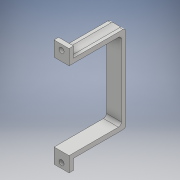
# Autodesk Inventor part: battery-bracket
Saved by Autodesk Inventor 2018 (Build 220112000, 112)
## iProperties
Created: 2017-10-22
Part Number: battery-bracket
Material: Generic
Document SubType Name: Modeling
Designer: leo2a
Density: 1 g/cm^3
Appearance: Default
Author: leo2a
Autodesk Inventor part; units mm, degrees
ref_plane "YZ Plane" through (0, 0, 0) normal (1, 0, 0) x (0, 1, 0)
ref_plane "XZ Plane" through (0, 0, 0) normal (0, 1, 0) x (-1, 0, 0)
ref_plane "XY Plane" through (0, 0, 0) normal (0, 0, 1) x (1, 0, 0)
sketch "Sketch1" plane through (0, 0, 0) normal (1, 0, 0) x (0, 1, 0)
  line L0 (0, 0) -> (0, 26)
  line L1 (0, 26) -> (-35, 26)
  line L2 (0, 0) -> (3, 0)
  line L3 (3, 0) -> (3, 29)
  line L4 (3, 29) -> (-32, 29)
  line L5 (-32, 29) -> (-32, 36)
  line L6 (-32, 36) -> (-35, 36)
  line L7 (-35, 36) -> (-35, 26)
  line L8 (0, 0) -> (0, -26)
  line L9 (0, -26) -> (-35, -26)
  line L10 (3, 0) -> (3, -29)
  line L11 (3, -29) -> (-32, -29)
  line L12 (-32, -29) -> (-32, -36)
  line L13 (-32, -36) -> (-35, -36)
  line L14 (-35, -36) -> (-35, -26)
  dimension "d0" = 26
  dimension "d1" = 35
  dimension "d2" = 3
  dimension "d3" = 29
  dimension "d4" = 35
  dimension "d5" = 7
  constraints: 30 end point, 6 perpendicular, 6 symmetric about line, 1 horizontal, 1 vertical
  measures "d0" distance of L0.start L0.end
  measures "d1" distance of L0.end L1.end
  measures "d2" distance of L0.start L2.end
  measures "d3" distance of L2.end L3.end
  measures "d4" distance of L3.end L4.end
  measures "d5" distance of L4.end L5.end
extrude "Extrusion1" add sketch "Sketch1" along normal blind 10
fillet "Fillet1" radius 2 4 edges at (5, 3, 29) (5, 0, 26) (5, 0, -26) (5, 3, -29)
sketch "Sketch2" plane through (0, -32, 36) normal (0, 1, 0) x (1, 0, 0)
  line L0 (0, 7) -> (0, 0) projected
  line L1 (0, 3.5) -> (5, 3.5)
  line L2 (0, 62) -> (0, 72) projected
  line L3 (0, 72) -> (0, 68.5)
  line L4 (0, 68.5) -> (5, 68.5)
  point P0 (0, 36)
  dimension "d9" = 3.5
  constraints: 6 end point, 2 coincident, 1 horizontal, 1 midpoint, 1 perpendicular, 1 point on line
  measures "d9" distance of L2.end L3.end
hole "Hole1" at (5, -32, 32.5) at (5, -32, -32.5) direction (0, -1, 0) diameter 3.4 end through all clearance for "Socket Head Cap Screw ISO 4762" size "M3" standard "ISO"
sketch "Sketch3" plane through (0, -32, 36) normal (0, 1, 0) x (1, 0, 0)
  circle A0 centre (5, 3.5) radius 1.7 projected
  circle A1 centre (5, 3.5) radius 4.5
  circle A2 centre (5, 68.5) radius 1.7 projected
  circle A3 centre (5, 68.5) radius 4.5
  point P0 (0, 36)
  dimension "d17" = 9
  dimension "d18" = 9
  constraints: 2 centre point, 2 coincident
  measures "d17" diameter of A1
  measures "d18" diameter of A3
extrude "Extrusion2" cut sketch "Sketch3" along normal through all
body "Solid1"
